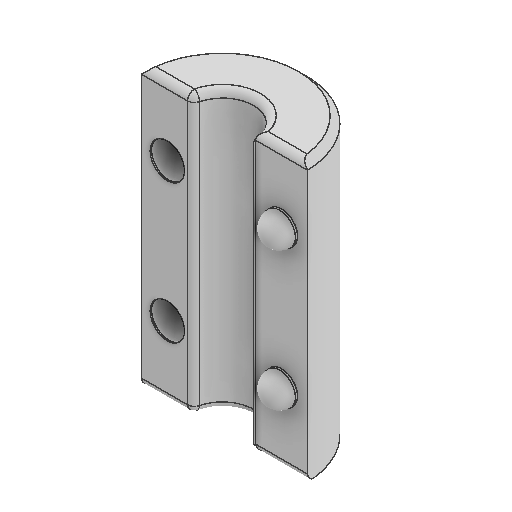
# Autodesk Inventor part: ucacheCableGlandAdapter
Saved by Autodesk Inventor 2025 (Build 290162000, 162)
## iProperties
Created: 2025-01-06
Part Number: ucacheCableGlandAdapter
Material: Generic
Document SubType Name: Modeling
Designer: derm
Density: 1 g/cm^3
Appearance: Default
Author: derm
Autodesk Inventor part; units mm, degrees
ref_plane "YZ Plane" through (0, 0, 0) normal (1, 0, 0) x (0, 1, 0)
ref_plane "XZ Plane" through (0, 0, 0) normal (0, 1, 0) x (-1, 0, 0)
ref_plane "XY Plane" through (0, 0, 0) normal (0, 0, 1) x (1, 0, 0)
sketch "Sketch1" plane through (0, 0, 0) normal (0, 0, 1) x (1, 0, 0)
  line L0 (0, 0) -> (0, 20)
  line L1 (0, 20) -> (2.25, 20)
  line L2 (2.25, 20) -> (2.25, 0)
  line L3 (2.25, 0) -> (0, 0)
  line L4 (0, 0) -> (0, 20)
  line L5 (0, 20) -> (6, 20)
  line L6 (6, 20) -> (6, 0)
  line L7 (6, 0) -> (0, 0)
  line L8 (0, 0) -> (0, 20)
  dimension "d0" = 2.25
  dimension "d1" = 6
  dimension "d2" = 20
  constraints: 18 end point, 4 parallel, 2 horizontal, 2 perpendicular, 1 vertical
  measures "d0" distance between parallel lines of L2 L0
  measures "d1" distance between parallel lines of L6 L0
  measures "d2" distance of L5.end L6.end
revolve "Revolution1" add sketch "Sketch1" angle 180 about axis through (0, 0, 0) along (0, 1, 0) contours L2 L5 L6 L7
sketch "Sketch2" plane through (2.25, 20, 0) normal (0, 0, 1) x (1, 0, 0)
  line L0 (3.75, 0) -> (0, 0) projected
  line L1 (0, 0) -> (0, -20) projected
  line L2 (0, -20) -> (3.75, -20) projected
  line L3 (3.75, -20) -> (3.75, 0) projected
  circle A0 centre (1.875, -5) radius 1.25
  circle A1 centre (1.875, -15) radius 1.25
  point P0 (-2.25, -20)
  dimension "d5" = 2.5
  dimension "d6" = 2.5
  dimension "d7" = 5
  dimension "d8" = 5
  constraints: 2 centre point
  measures "d5" diameter of A1
  measures "d6" diameter of A0
  measures "d7" distance from line of L2 A1.centre
  measures "d8" distance from line of L0 A0.centre
extrude "Extrusion1" add sketch "Sketch2" along normal blind 1.25 contours A0 | A1
fillet "Fillet1" radius 1.25 2 edges at (2.875, 15, 1.25) (2.875, 5, 1.25)
sketch "Sketch3" plane through (-6, 20, 0) normal (0, 0, 1) x (1, 0, 0)
  line L0 (12, 0) -> (8.25, 0) projected
  line L1 (8.25, 0) -> (8.25, -20) projected
  line L2 (8.25, -20) -> (12, -20) projected
  line L3 (12, -20) -> (12, 0) projected
  line L4 (3.75, 0) -> (0, 0) projected
  line L5 (0, 0) -> (0, -20) projected
  line L6 (0, -20) -> (3.75, -20) projected
  line L7 (3.75, -20) -> (3.75, 0) projected
  circle A0 centre (1.875, -4.9722) radius 1.25
  circle A1 centre (1.875, -14.9821) radius 1.25
  point P0 (6, -20)
  dimension "d12" = 2.5
  constraints: 2 centre point
  measures "d12" diameter of A0
extrude "Extrusion2" cut sketch "Sketch3" against normal blind 1.5 contours A0 | A1
fillet "Fillet2" radius 1.25 2 edges at (-5.375, 15.0278, -1.5) (-5.375, 5.0179, -1.5)
thicken "Thicken1" operation cut thickness 0.1 both sides no extend neighbours no toward (-0.9967573, 0.0804666, 0) faces at (5.3709, 14.8994, 0.0001) (4.5529, 16.1596, 0.1864) (4.125, 15, 1.25)
thicken "Thicken2" operation cut thickness 0.1 both sides no extend neighbours no toward (-0.9870503, 0.1604113, 0) faces at (5.3588, 4.7995, 0) (3.6971, 3.8404, 0.1864) (4.125, 5, 1.25)
chamfer "Chamfer1" distance 0.5 angle 45 1 edges at (0, 20, -6)
sketch "Sketch4" plane through (-6, 0, 0) normal (0, 0, 1) x (1, 0, 0)
  circle A0 centre (1.875, 15.0278) radius 1.25 projected
  circle A1 centre (1.875, 5.0179) radius 1.25 projected
  line L0 (0, 19.5) -> (0.5, 20) projected
  line L1 (0, 19.5) -> (0, 0) projected
  line L2 (0, 0) -> (3.75, 0) projected
  line L3 (3.75, 20) -> (0.5, 20) projected
  line L4 (11.5, 20) -> (12, 19.5) projected
  line L5 (11.5, 20) -> (8.25, 20) projected
  line L6 (8.25, 0) -> (12, 0) projected
  line L7 (12, 0) -> (12, 19.5) projected
  circle A2 centre (10.125, 5) radius 1.15 projected
  circle A3 centre (10.125, 15) radius 1.15 projected
  line L8 (3.0582, 20) -> (7.9418, 20)
  line L9 (7.9418, 20) -> (7.9418, 0)
  line L10 (7.9418, 0) -> (3.0582, 0)
  line L11 (3.0582, 0) -> (3.0582, 20)
  line L12 (8.25, 20) -> (8.25, 0) projected
  line L13 (3.75, 0) -> (3.75, 20) projected
  point P0 (6, 0)
  point P1 (3.0582, 0)
  point P2 (7.9418, 20)
  point P3 (7.9418, 0)
  point P4 (3.75, 0)
  point P5 (7.75, 0)
  point P6 (7.75, 20)
  point P7 (7.9418, 0)
  constraints: 8 end point, 2 parallel, 1 horizontal, 1 perpendicular
extrude "Extrusion3" cut sketch "Sketch4" against normal blind 0.15 contours A0 L11 L3 L13 L2 A1 | A0 L11 A1 L2 L1 L0 L3 | L8 L9 L10 L13 | L4 L7 L6 L12 L5
fillet "Fillet4" radius 0.5 1 edges at (-2.245, 10, -0.15)
fillet "Fillet5" radius 0.5 8 edges at (-4.085, 20, -0.15) (-2.3631, 20, -0.2569) (3.874, 20, -0.15) (0.2678, 20, -2.234) (-4.3351, 0, -0.15) (-2.3631, 0, -0.2569) (4.1241, 0, -0.15) (0.2678, 0, -2.234)
body "Solid1"
